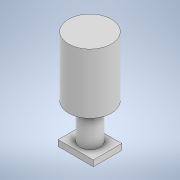
# Autodesk Inventor part: 警示燈
Saved by Autodesk Inventor 2022 (Build 260153000, 153)
## iProperties
Created: 2023-03-12
Part Number: 警示燈
Material: 一般
Document SubType Name: Modeling
Designer: User
Mass: 1436.93 g
Surface Area: 883.134 cm^2
Volume: 1436.93 cm^3
Density: 1 g/cm^3
Appearance: 預設
Author: User
Autodesk Inventor part; units mm, degrees
ref_plane "YZ Plane" through (0, 0, 0) normal (1, 0, 0) x (0, 1, 0)
ref_plane "XZ Plane" through (0, 0, 0) normal (0, 1, 0) x (-1, 0, 0)
ref_plane "XY Plane" through (0, 0, 0) normal (0, 0, 1) x (1, 0, 0)
sketch "草圖1" plane through (0, 0, 0) normal (0, 0, 1) x (1, 0, 0)
  line L0 (-10.2978, 0) -> (61.7865, 0) construction
  line L1 (0, -46.4493) -> (0, 291.2466) construction
  line L2 (0, 243.0043) -> (51.4888, 243.0043)
  line L3 (51.4888, 243.0043) -> (51.4888, 99.1203)
  line L4 (51.4888, 99.1203) -> (0, 99.1203)
  line L5 (0, 99.1203) -> (0, 243.0043)
  line L6 (0, 99.1203) -> (24.2134, 99.1203)
  line L7 (24.2134, 99.1203) -> (24.2134, 1.7929)
  line L8 (24.2134, 1.7929) -> (0, 1.7929)
  line L9 (0, 1.7929) -> (0, 99.1203)
  constraints: 16 end point, 4 parallel, 2 horizontal, 2 perpendicular, 1 point on line
revolve "迴轉1" add sketch "草圖1" angle 360 about axis through (0, 99.1203, 0) along (0, 1, 0)
sketch "草圖2" plane through (0, 0, 0) normal (0, 1, 0) x (-1, 0, 0)
  line L0 (42.1711, -34.1557) -> (-42.1711, -34.1557)
  line L1 (-42.1711, -34.1557) -> (-42.1711, 34.1557)
  line L2 (-42.1711, 34.1557) -> (42.1711, 34.1557)
  line L3 (42.1711, 34.1557) -> (42.1711, -34.1557)
  line L4 (59.0396, 0) -> (-59.0396, 0) construction
  line L5 (0, -47.818) -> (0, 47.818) construction
  point P0 (0, 0)
  constraints: 8 end point, 2 parallel, 1 horizontal, 1 perpendicular, 2 other
extrude "擠出1" add sketch "草圖2" along normal blind 14.2875
